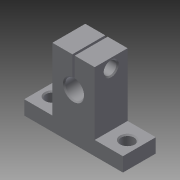
# Autodesk Inventor part: Linear Rail Shaft Guide
Saved by Autodesk Inventor 2015 SP1 (Build 190203100, 203)
## iProperties
Created: 2015-02-20
Part Number: Linear Rail Shaft Guide
Material: Generic
Document SubType Name: Modeling
Designer: pltwe4
Density: 1 g/cm^3
Appearance: Default
Author: pltwe4
Autodesk Inventor part; units mm, degrees
ref_plane "YZ Plane" through (0, 0, 0) normal (1, 0, 0) x (0, 1, 0)
ref_plane "XZ Plane" through (0, 0, 0) normal (0, 1, 0) x (-1, 0, 0)
ref_plane "XY Plane" through (0, 0, 0) normal (0, 0, 1) x (1, 0, 0)
sketch "Sketch1" plane through (0, 0, 0) normal (0, 0, 1) x (1, 0, 0)
  line L0 (0, 39.36) -> (0, -6.56) projected
  line L1 (-29.4, 0) -> (29.4, 0) projected
  line L2 (-21, 0) -> (21, 0)
  line L3 (21, 0) -> (21, 6)
  line L4 (21, 6) -> (9, 6)
  line L5 (9, 6) -> (9, 32.8)
  line L6 (9, 32.8) -> (0.5, 32.8)
  line L7 (0.5, 32.8) -> (0.5, 23.9686)
  line L8 (-0.5, 23.9686) -> (-0.5, 32.8)
  line L9 (-0.5, 32.8) -> (-9, 32.8)
  line L10 (-9, 32.8) -> (-9, 6)
  line L11 (-9, 6) -> (-21, 6)
  line L12 (-21, 6) -> (-21, 0)
  circle A0 centre (0, 20) radius 4
  point P0 (0, 0)
  dimension "d0" = 42
  dimension "d1" = 6
  dimension "d2" = 20
  dimension "d3" = 32.8
  dimension "d4" = 21
  dimension "d5" = 18
  dimension "d6" = 8
  dimension "d7" = 1
  constraints: 22 end point, 8 perpendicular, 3 point on line, 2 point on circle, 1 centre point, 1 parallel, 1 vertical, 5 other
  measures "d0" distance between parallel lines of L3 L12
  measures "d1" distance between parallel lines of L1 L11
  measures "d2" distance from line of L1 A0.centre
  measures "d3" distance between parallel lines of L1 L6
  measures "d4" distance from line of L12 A0.centre
  measures "d5" distance between parallel lines of L5 L10
  measures "d6" diameter of A0
  measures "d7" distance between parallel lines of L8 L7
extrude "Extrusion1" add sketch "Sketch1" along normal mid plane 14 contours A0 L7 L6 L5 L4 L3 L1 L0 | L0 L1 L12 L11 L10 L9 L8 A0
sketch "Sketch2" plane through (-21, 6, -7) normal (0, 1, 0) x (1, 0, 0)
  line L0 (0, 0) -> (12, 0) projected
  line L1 (0, 0) -> (0, -14) projected
  line L2 (12, -14) -> (0, -14) projected
  line L3 (12, 0) -> (12, -14) projected
  line L4 (30, 0) -> (42, 0) projected
  line L5 (30, 0) -> (30, -14) projected
  line L6 (42, -14) -> (30, -14) projected
  line L7 (42, 0) -> (42, -14) projected
  circle A0 centre (5, -7) radius 2.75
  circle A1 centre (37, -7) radius 2.75
  line L8 (21, 2.8) -> (21, -16.8) projected
  line L9 (50.4, -7) -> (-8.4, -7) projected
  point P0 (21, -7)
  dimension "d10" = 5.5
  dimension "d11" = 32
  constraints: 2 centre point, 1 point on line, 1 other
  measures "d10" diameter of A0
  measures "d11" distance of A1.centre A0.centre
extrude "Extrusion2" cut sketch "Sketch2" against normal up to next contours L9 A0 | A0 L9 | L9 A1 | A1 L9
sketch "Sketch3" plane through (9, 6, 7) normal (1, 0, 0) x (0, 0, -1)
  line L0 (14, 26.8) -> (0, 26.8) projected
  line L1 (0, 0) -> (0, 26.8) projected
  line L2 (14, 0) -> (0, 0) projected
  line L3 (14, 26.8) -> (14, 0) projected
  circle A0 centre (7, 22.8) radius 2.75
  line L4 (14, 26.8) -> (0, 26.8) construction
  line L5 (7, 26.8) -> (7, 0) construction
  line L6 (14, 0) -> (0, 0) construction
  point P0 (7, -6)
  dimension "d14" = 5.5
  dimension "d15" = 4
  constraints: 2 end point, 2 midpoint, 1 centre point, 1 point on line
  measures "d14" diameter of A0
  measures "d15" distance from line of L0 A0.centre
extrude "Extrusion3" cut sketch "Sketch3" against normal up to surface (18 mm away) contours A0
chamfer "Chamfer1" distance 0.5 angle 45 6 edges at (0, 16, 7) (0, 16, -7) (9, 28.8, 2.75) (13.25, 6, 0) (-9, 28.8, 2.75) (-18.75, 6, 0)
body "Solid1"
